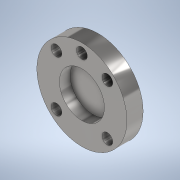
# Autodesk Inventor part: flancheDeMontaje
Saved by Autodesk Inventor 2021.5 (Build 255421000, 421)
## iProperties
Created: 2024-11-17
Part Number: flancheDeMontaje
Material: Genérico
Document SubType Name: Modeling
Designer: Joho_
Density: 1 g/cm^3
Appearance: Valor por defecto
Author: Joho_
Autodesk Inventor part; units mm, degrees
ref_plane "YZ Plane" through (0, 0, 0) normal (1, 0, 0) x (0, 1, 0)
ref_plane "XZ Plane" through (0, 0, 0) normal (0, 1, 0) x (-1, 0, 0)
ref_plane "XY Plane" through (0, 0, 0) normal (0, 0, 1) x (1, 0, 0)
sketch "Boceto1" plane through (0, 0, 0) normal (0, 0, 1) x (1, 0, 0)
  circle A0 centre (0, 0) radius 25
  circle A1 centre (0, 0) radius 20
  line L0 (0, 0) -> (14.1421, 14.1421)
  line L1 (0, 0) -> (20, 0) construction
  circle A2 centre (14.1421, 14.1421) radius 3
  circle A3 centre (14.1421, -14.1421) radius 3
  circle A4 centre (0, 0) radius 20
  circle A5 centre (-14.1421, -14.1421) radius 3
  circle A6 centre (0, 0) radius 20
  circle A7 centre (-14.1421, 14.1421) radius 3
  circle A8 centre (0, 0) radius 20
  circle A9 centre (0, 20) radius 3
  circle A10 centre (0, 0) radius 12.5
  dimension "d1" = 40
  dimension "d0" = 50
  dimension "d2" = 45
  dimension "d3" = 6
  dimension "d6" = 360
  dimension "d8" = 6
  dimension "d9" = 25
  constraints: 9 coincident, 8 centre point, 4 end point, 2 coincident with centre, 2 point on circle, 1 equal length, 1 horizontal, 26 other
  measures "d0" diameter of A0
  measures "d2" angle of L1 L0
  measures "d3" diameter of A2
  measures "d8" diameter of A9
  measures "d9" diameter of A10
extrude "Extrusión1" add sketch "Boceto1" along normal blind 9 contours A0 | A1 A3 A5 A7 A9 A2
extrude "Extrusión2" add sketch "Boceto1" along normal blind 3 contours A10
